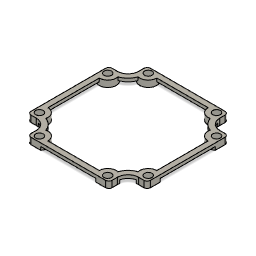
stepper_spacer (Autodesk Fusion 360 design; units mm, degrees)
Autodesk Fusion 360 part; units mm, degrees
sketch "Sketch1" plane through (0, 0, 0) normal (0, 1, 0) x (1, 0, 0)
  line L0 (-28, 17.5) -> (-28, 0)
  line L1 (-20.4645, 20.4645) -> (0, 0) construction
  line L2 (-28, 0) -> (0, 0) construction
  line L3 (-26.5, 19) -> (-24, 19)
  arc A0 (-24, 19) -> (-20.4645, 20.4645) centre (-24, 24) ccw
  line L4 (-20.4645, 20.4645) -> (-40.9289, 0) construction
  circle A1 centre (-25.5, 16) radius 1.75
  circle A2 centre (-25.5, 16) radius 4
  arc A3 (-26.5, 19) -> (-28, 17.5) centre (-26.5, 17.5) ccw
  arc A4 (-24, 16.5) -> (-18.6967, 18.6967) centre (-24, 24) ccw
  line L5 (-25.5, 16.5) -> (-24, 16.5)
  line L6 (-25.5, 16.5) -> (-25.5, 0)
  circle A5 centre (-16, 25.5) radius 1.75
  circle A6 centre (-16, 25.5) radius 4
  arc A7 (-20.4645, 20.4645) -> (-19, 24) centre (-24, 24) ccw
  line L7 (-19, 26.5) -> (-19, 24)
  arc A8 (-17.5, 28) -> (-19, 26.5) centre (-17.5, 26.5) ccw
  line L8 (-17.5, 28) -> (0, 28)
  line L9 (-16.5, 25.5) -> (0, 25.5)
  line L10 (-16.5, 25.5) -> (-16.5, 24)
  arc A9 (-18.6967, 18.6967) -> (-16.5, 24) centre (-24, 24) ccw
  circle A10 centre (-25.5, -16) radius 4
  arc A11 (-19, -26.5) -> (-17.5, -28) centre (-17.5, -26.5) ccw
  arc A12 (-19, -24) -> (-20.4645, -20.4645) centre (-24, -24) ccw
  arc A13 (-20.4645, -20.4645) -> (-24, -19) centre (-24, -24) ccw
  line L11 (-25.5, -16.5) -> (-25.5, 0)
  circle A14 centre (-16, -25.5) radius 4
  arc A15 (-18.6967, -18.6967) -> (-24, -16.5) centre (-24, -24) ccw
  line L12 (-16.5, -25.5) -> (0, -25.5)
  line L13 (-28, -17.5) -> (-28, 0)
  line L14 (-26.5, -19) -> (-24, -19)
  line L15 (-17.5, -28) -> (0, -28)
  arc A16 (-28, -17.5) -> (-26.5, -19) centre (-26.5, -17.5) ccw
  line L16 (-19, -26.5) -> (-19, -24)
  circle A17 centre (-16, -25.5) radius 1.75
  circle A18 centre (-25.5, -16) radius 1.75
  arc A19 (-16.5, -24) -> (-18.6967, -18.6967) centre (-24, -24) ccw
  line L17 (-25.5, -16.5) -> (-24, -16.5)
  line L18 (-16.5, -25.5) -> (-16.5, -24)
  line L19 (0, 28) -> (0, -28) construction
  line L20 (25.5, -16.5) -> (25.5, 0)
  line L21 (25.5, -16.5) -> (24, -16.5)
  arc A20 (26.5, -19) -> (28, -17.5) centre (26.5, -17.5) ccw
  line L22 (16.5, 25.5) -> (0, 25.5)
  line L23 (17.5, -28) -> (0, -28)
  line L24 (28, 0) -> (0, 0) construction
  line L25 (25.5, 16.5) -> (25.5, 0)
  arc A21 (28, 17.5) -> (26.5, 19) centre (26.5, 17.5) ccw
  arc A22 (18.6967, 18.6967) -> (24, 16.5) centre (24, 24) ccw
  line L26 (20.4645, 20.4645) -> (0, 0) construction
  circle A23 centre (16, 25.5) radius 1.75
  line L27 (17.5, 28) -> (0, 28)
  circle A24 centre (25.5, 16) radius 1.75
  arc A25 (19, 24) -> (20.4645, 20.4645) centre (24, 24) ccw
  line L28 (16.5, -25.5) -> (16.5, -24)
  line L29 (28, 17.5) -> (28, 0)
  line L30 (16.5, 25.5) -> (16.5, 24)
  line L31 (28, -17.5) -> (28, 0)
  arc A26 (17.5, -28) -> (19, -26.5) centre (17.5, -26.5) ccw
  arc A27 (24, -19) -> (20.4645, -20.4645) centre (24, -24) ccw
  circle A28 centre (25.5, 16) radius 4
  circle A29 centre (16, 25.5) radius 4
  arc A30 (20.4645, 20.4645) -> (24, 19) centre (24, 24) ccw
  line L32 (26.5, 19) -> (24, 19)
  arc A31 (24, -16.5) -> (18.6967, -18.6967) centre (24, -24) ccw
  circle A32 centre (16, -25.5) radius 1.75
  line L33 (25.5, 16.5) -> (24, 16.5)
  circle A33 centre (25.5, -16) radius 1.75
  line L34 (19, -26.5) -> (19, -24)
  line L35 (16.5, -25.5) -> (0, -25.5)
  line L36 (19, 26.5) -> (19, 24)
  arc A34 (18.6967, -18.6967) -> (16.5, -24) centre (24, -24) ccw
  circle A35 centre (25.5, -16) radius 4
  arc A36 (16.5, 24) -> (18.6967, 18.6967) centre (24, 24) ccw
  circle A37 centre (16, -25.5) radius 4
  arc A38 (19, 26.5) -> (17.5, 28) centre (17.5, 26.5) ccw
  arc A39 (20.4645, -20.4645) -> (19, -24) centre (24, -24) ccw
  line L37 (26.5, -19) -> (24, -19)
  point P0 (-28, 19)
  point P1 (-20.4645, 20.4645)
  point P2 (23.8544, 0)
  point P3 (23.8544, 0)
  point P4 (23.8544, 0)
  point P5 (-20.4645, 20.4645)
  point P6 (-19, 28)
  point P7 (-20.4645, 20.4645)
  point P8 (-20.4645, -20.4645)
  point P9 (23.8544, 0)
  point P10 (-20.4645, -20.4645)
  point P11 (-19, -28)
  point P12 (23.8544, 0)
  point P13 (23.8544, 0)
  point P14 (11.9272, -28.2627)
  point P15 (-20.4645, -20.4645)
  point P16 (-20.4645, -20.4645)
  point P17 (-28, -19)
  point P18 (19, -28)
  point P19 (20.4645, 20.4645)
  point P20 (20.4645, -20.4645)
  point P21 (20.4645, 20.4645)
  point P22 (20.4645, 20.4645)
  point P23 (19, 28)
  point P24 (28, -19)
  point P25 (20.4645, -20.4645)
  point P26 (20.4645, -20.4645)
  point P27 (20.4645, -20.4645)
  point P28 (28, 19)
  dimension "d1" = 45
  dimension "d2" = 19
  dimension "d3" = 4
  dimension "d4" = 5
  dimension "d5" = 2.5
  dimension "d6" = 3
  dimension "d7" = 3.5
  dimension "d13" = 1.5
  dimension "d18" = 8
  dimension "d19" = 2.5
  constraint vertical L0
  constraint coincident L1.end L2.end
  constraint perpendicular L0 L2
  constraint perpendicular L0 L3
  constraint tangent L3 A0
  constraint perpendicular L1 L4
  constraint coincident P7 P5
  constraint tangent A0 L4
  constraint coincident L2 L4.end
  constraint concentric A1 A2
  constraint coincident P0 L3
  constraint coincident P0 L0
  constraint tangent L3 A3
  constraint tangent L0 A3
  constraint symmetric P7 L1 P5
  constraint symmetric L1.end L2 L24.end
  constraint symmetric P0 L1 P6
  constraint symmetric L0.end L1 L8.end
  constraint symmetric L1 L3.end A7.end
  constraint symmetric L1 P7 P5
  constraint symmetric L1 A0 A7
  constraint symmetric L1 A1 A5
  constraint symmetric L1 A2 A6
  constraint symmetric L1 L3.start L7.start
  constraint symmetric L1 L0.start A8.start
  constraint symmetric L1 A3 A8
  constraint symmetric L1 A4.end A9.start
  constraint symmetric L1 A4.start L10.end
  constraint symmetric L1 A4 A9
  constraint symmetric L1 L5.start L9.start
  constraint symmetric L1 L6.end L9.end
  constraint symmetric P0 L2 P17
  constraint symmetric L0.end L2 L13.end
  constraint symmetric P7 L2 P16
  constraint symmetric L2 L3.end A13.end
  constraint symmetric L2 P7 P16
  constraint symmetric L2 A0 A13
  constraint symmetric L2 A1 A18
  constraint symmetric L2 A2 A10
  constraint symmetric L2 L3.start L14.start
  constraint symmetric L2 L0.start L13.start
  constraint symmetric L2 A3 A16
  constraint symmetric L2 L1.end L24.end
  constraint symmetric L2 P13 P12
  constraint symmetric L2 A4.end A15.start
  constraint symmetric L2 A4.start A15.end
  constraint symmetric L2 A4 A15
  constraint symmetric L2 L5.start L11.start
  constraint symmetric L2 L6.end L11.end
  constraint symmetric L2 P6 P11
  constraint symmetric L2 L8.end L15.end
  constraint symmetric L2 A7.end A12.start
  constraint symmetric L2 L7.start A11.start
  constraint symmetric L2 A8.start A11.end
  constraint symmetric L2 L9.end L12.end
  constraint symmetric L2 L9.start L12.start
  constraint symmetric L2 L10.end A19.start
  constraint symmetric L2 A5 A17
  constraint symmetric L2 A6 A14
  constraint symmetric L2 A7 A12
  constraint symmetric L2 A8 A11
  constraint symmetric L2 A9 A19
  constraint symmetric P0 L19 P28
  constraint symmetric L0.end L19 L24.start
  constraint symmetric P7 L19 P22
  constraint symmetric L1.end L19 L2.end
  constraint symmetric L3.end L19 A30.end
  constraint symmetric A0 L19 A30
  constraint symmetric A1 L19 A24
  constraint symmetric A2 L19 A28
  constraint symmetric L3.start L19 A21.end
  constraint symmetric L0.start L19 A21.start
  constraint symmetric A3 L19 A21
  constraint symmetric A4.end L19 A22.start
  constraint symmetric A4.start L19 A22.end
  constraint symmetric A4 L19 A22
  constraint symmetric L5.start L19 L25.start
  constraint symmetric L6.end L19 L20.end
  constraint symmetric P6 L19 P23
  constraint symmetric L8.end L19 L27.end
  constraint symmetric A7.end L19 A25.start
  constraint symmetric L7.start L19 L36.start
  constraint symmetric A8.start L19 L27.start
  constraint symmetric L9.end L19 L22.end
  constraint symmetric L9.start L19 L22.start
  constraint symmetric L10.end L19 L30.end
  constraint symmetric A5 L19 A23
  constraint symmetric A6 L19 A29
  constraint symmetric A7 L19 A25
  constraint symmetric A8 L19 A38
  constraint symmetric A9 L19 A36
  constraint symmetric A13.end L19 A27.start
  constraint symmetric P16 L19 P27
  constraint symmetric A15.end L19 L21.end
  constraint symmetric L11.start L19 L20.start
  constraint symmetric P11 L19 P18
  constraint symmetric A12.start L19 L34.end
  constraint symmetric A19.start L19 L28.end
  constraint symmetric L13.start L19 A20.end
  constraint symmetric L14.start L19 A20.start
  constraint symmetric A15.start L19 A31.end
  constraint symmetric L12.start L19 L28.start
  constraint symmetric A11.end L19 L23.start
  constraint symmetric A11.start L19 A26.end
  constraint symmetric L12.end L19 L35.end
  constraint symmetric L15.end L19 L23.end
  constraint symmetric P17 L19 P24
  constraint symmetric A10 L19 A35
  constraint symmetric A11 L19 A26
  constraint symmetric A12 L19 A39
  constraint symmetric A13 L19 A27
  constraint symmetric A14 L19 A37
  constraint symmetric A15 L19 A31
  constraint symmetric A16 L19 A20
  constraint symmetric A17 L19 A32
  constraint symmetric A18 L19 A33
  constraint symmetric A19 L19 A34
  measures "d1" angle of L1 L2
  measures "d2" distance of P0 L0.end
  measures "d3" distance of P0 L3.end
  measures "d4" radius of A0
  measures "d5" distance of L0 A1.centre
  measures "d6" distance of L3 A1.centre
  measures "d7" diameter of A1
  measures "d13" radius of A3
  measures "d18" diameter of A2
extrude "Extrude1" add sketch "Sketch1" along normal blind 1.5 contours L0 L3 A0 A1 A2 A3 A4 L6 | L0 A2 L6 A10 L11 L13 | A0 A2 A4 A6 A7 A9 | A1 A2 A4 L6 | A10 A13 L11 A15 L13 L14 A16 A18 | A10 L11 A15 A18 | A10 A12 A13 A14 A15 A19 | A5 A6 A7 L7 A8 L8 L9 A9 | A6 L8 L9 L22 L27 A29 | A5 A6 L9 A9 | A11 A12 A14 L12 L15 L16 A17 A19 | A14 L12 A17 A19 | A14 L12 L15 L23 L35 A37 | L22 A23 L27 A25 A29 L36 A36 A38 | L22 A23 A29 A36 | L23 A26 A32 L34 L35 A34 A37 A39 | A22 A25 A28 A29 A30 A36 | A32 L35 A34 A37 | A27 A31 A34 A35 A37 A39 | L25 A21 A22 A24 L29 A28 A30 L32 | L25 A22 A24 A28 | L20 L25 L29 L31 A28 A35 | L20 A31 A33 A35 | L20 A20 L31 A27 A31 A33 A35 L37
extrude "Extrude2" add sketch "Sketch1" against normal blind 1.5 contours L0 L3 A0 A1 A2 A3 A4 L6 | A1 A2 A4 L6 | A10 A13 L11 A15 L13 L14 A16 A18 | A10 L11 A15 A18 | A5 A6 A7 L7 A8 L8 L9 A9 | A5 A6 L9 A9 | A11 A12 A14 L12 L15 L16 A17 A19 | A14 L12 A17 A19 | L22 A23 L27 A25 A29 L36 A36 A38 | L22 A23 A29 A36 | L23 A26 A32 L34 L35 A34 A37 A39 | A32 L35 A34 A37 | L25 A21 A22 A24 L29 A28 A30 L32 | L25 A22 A24 A28 | L20 A31 A33 A35 | L20 A20 L31 A27 A31 A33 A35 L37
